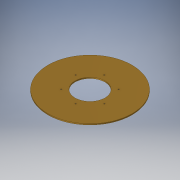
# Autodesk Inventor part: 4K shield bottom
Saved by Autodesk Inventor 2018 (Build 220112000, 112)
## iProperties
Created: 2019-03-11
Part Number: 4K shield bottom
Material: Brass, Soft Yellow
Document SubType Name: Modeling
Designer: Admin
Density: 8.47 g/cm^3
Appearance: Brass - Satin
Author: Admin
Autodesk Inventor part; units mm, degrees
ref_plane "YZ Plane" through (0, 0, 0) normal (1, 0, 0) x (0, 1, 0)
ref_plane "XZ Plane" through (0, 0, 0) normal (0, 1, 0) x (-1, 0, 0)
ref_plane "XY Plane" through (0, 0, 0) normal (0, 0, 1) x (1, 0, 0)
sketch "Sketch1" plane through (0, 0, 0) normal (0, 1, 0) x (-1, 0, 0)
  circle A0 centre (0, 0) radius 98.425
  circle A1 centre (0, 0) radius 34.925
  dimension "d0" = 196.85
  dimension "d1" = 63.5
  constraints: 2 centre point, 2 coincident
  measures "d0" diameter of A0
  measures "d1" radial gap between concentric circles of A1 A0
extrude "Extrusion1" add sketch "Sketch1" along normal blind 2.54
sketch "Sketch2" plane through (0, 2.54, 0) normal (0, 1, 0) x (1, 0, 0)
  line L0 (0, 0) -> (33.676, 33.676) construction
  line L1 (0, 0) -> (47.625, 0) construction
  dimension "d4" = 47.625
  dimension "d5" = 45
  constraints: 4 end point, 1 coincident, 1 equal length, 1 horizontal
  measures "d4" distance of L0.start L0.end
  measures "d5" angle of L1 L0
hole "Hole1" at (33.676, 2.54, -33.676) direction (0, -1, 0) diameter 2.8448 end through all
pattern_circular "Circular Pattern1" count 6 over 360 about axis through (0, 0, 0) along (0, 1, 0) of "Hole1"
body "Solid1"
